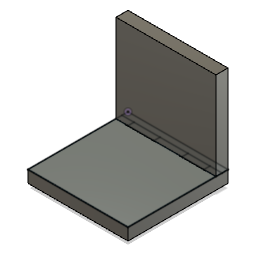
long tenons v2 (Autodesk Fusion 360 design; units mm, degrees)
Autodesk Fusion 360 part; units mm, degrees
sketch "Sketch1" plane through (0, 0, 0) normal (0, 1, 0) x (1, 0, 0)
  line L0 (0, 0) -> (25, 0)
  line L1 (25, 0) -> (25, -25)
  line L2 (25, -25) -> (0, -25)
  line L3 (0, -25) -> (0, 0)
  line L4 (0, -3) -> (25, -3)
  line L5 (0, -1.5) -> (25, -1.5)
  line L6 (3, -1.5) -> (3, -3)
  line L7 (9.5, -1.5) -> (9.5, -3)
  line L8 (16.5, -1.5) -> (16.5, -3)
  line L9 (22, -1.5) -> (22, -3)
  dimension "d1" = 25
  dimension "d2" = 25
  dimension "d3" = 3
  dimension "d4" = 1.5
  dimension "d5" = 3
  dimension "d6" = 3
  dimension "d7" = 7
  dimension "d8" = 5.5
  constraint horizontal L0
  constraint vertical L1
  constraint horizontal L2
  constraint vertical L3
  constraint coincident L0.start L3.end
  constraint coincident L3 L4.start
  constraint coincident L1 L4.end
  constraint perpendicular L1 L4
  constraint coincident L3 L5.start
  constraint coincident L1 L5.end
  constraint perpendicular L1 L5
  constraint coincident L5 L6.start
  constraint coincident L4 L6.end
  constraint perpendicular L4 L6
  constraint coincident L5 L7.start
  constraint coincident L4 L7.end
  constraint perpendicular L4 L7
  constraint coincident L5 L8.start
  constraint coincident L4 L8.end
  constraint perpendicular L4 L8
  constraint coincident L5 L9.start
  constraint coincident L4 L9.end
  constraint perpendicular L4 L9
  measures "d1" distance of L0.start L0.end
  measures "d2" distance of L0.start L2.end
  measures "d3" distance of L0 L4
  measures "d4" distance of L4 L5
  measures "d5" distance of L1 L9
  measures "d6" distance of L3 L6
  measures "d7" distance of L7 L8
  measures "d8" distance of L8 L9
extrude "Extrude1" add sketch "Sketch1" against normal blind 3 contours L0 L1 L3 L5 | L3 L4 L5 L6 | L1 L4 L5 L9 | L1 L2 L3 L4 | L4 L5 L7 L8 makes body 1
extrude "Extrude2" add sketch "Sketch1" along normal blind 22 separate body contours L0 L1 L3 L5 | L3 L4 L5 L6 | L1 L4 L5 L9 | L4 L5 L6 L7 | L4 L5 L8 L9 | L4 L5 L7 L8 makes body 2
extrude "Extrude3" add sketch "Sketch1" against normal blind 4 contours L4 L5 L6 L7 | L4 L5 L8 L9 bodies 2
move_face "OffsetFaces1" offset -0.1 8 faces at (18.3333, -1, 1.5) (16.5, -1, 2) (5.1667, -1, 1.5) (3, -1, 2) (5.1667, -1, 3) (18.3333, -1, 3) (22, -1, 2) (9.5, -1, 2) on bodies 1
chamfer "Chamfer1" distance 0.5 angle 45 4 edges at (22.1, 0, 2.25) (16.4, 0, 2.25) (9.6, 0, 2.25) (2.9, 0, 2.25) on bodies 1
chamfer "Chamfer2" distance 1 angle 45 8 edges at (6.25, -3, 3.1) (6.25, -3, 1.4) (9.6, -3, 2.25) (2.9, -3, 2.25) (16.4, -3, 2.25) (19.25, -3, 3.1) (19.25, -3, 1.4) (22.1, -3, 2.25) on bodies 1
named bodies: "long tenons holes", "long tenons pegs"
